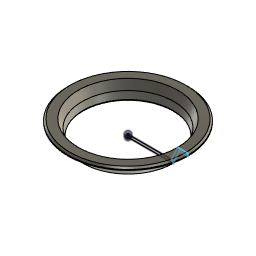
E2.2_TDP_TUTORIAL1 v1 (Autodesk Fusion 360 design; units mm, degrees)
Autodesk Fusion 360 part; units mm, degrees
sketch "Sketch1" plane through (0, 0, 0) normal (0, 1, 0) x (1, 0, 0)
  line L0 (0, 0) -> (52.0778, 0)
  line L1 (52.0778, 0) -> (59.2706, -16)
  line L2 (59.2706, -16) -> (71.3705, -16)
  line L3 (0, 3) -> (54.0184, 3)
  line L4 (54.0184, 3) -> (61.2112, -13)
  line L5 (61.2112, -13) -> (71.3705, -13)
  line L6 (71.3705, -16) -> (71.3705, -13)
  line L7 (52.0778, 0) -> (54.0184, 3)
  dimension "d1" = -3
  constraint coincident L0.start origin
  constraint horizontal L0
  constraint parallel L0 L2
revolve "Revolve1" add sketch "Sketch1" angle 360 about axis through (0, 0, 1.75) along (0, 0, 1)
chamfer "Chamfer1" distance 2 distance2 7 1 edges at (-48.5536, -18.8321, 0) measured on face at (53.1063, -5.3141, -2)
chamfer "Chamfer2" distance 2 distance2 2 1 edges at (-66.5407, -25.8087, 16) measured on face at (67.0715, -3.5457, 16)
chamfer "Chamfer3" distance 8 distance2 8 1 edges at (-57.0689, -22.1349, 13) measured on face at (67.7183, -3.5457, 13)
